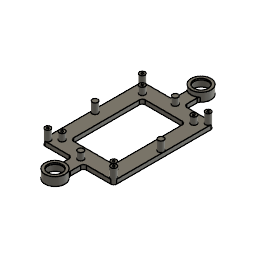
Waterproof box inset (Autodesk Fusion 360 design; units mm, degrees)
Autodesk Fusion 360 part; units mm, degrees
note: some values were not read from the file. Set by a fixed rule: which sketch regions a step uses.
sketch "Sketch1" plane through (0, 0, 0) normal (0, 1, 0) x (1, 0, 0)
  line L0 (0, 0) -> (-50, 0)
  line L1 (-50, 0) -> (-50, 70)
  line L2 (-50, 70) -> (0, 70)
  line L3 (0, 70) -> (0, 0)
  line L4 (-50, 0) -> (-48, 0)
  line L5 (-48, 0) -> (-48, 2)
  line L6 (-48, 2) -> (-50, 2)
  line L7 (-50, 2) -> (-50, 0)
  circle A0 centre (-48, 2) radius 2
  circle A1 centre (-48, 68) radius 2
  circle A2 centre (-2, 68) radius 2
  circle A3 centre (-2, 2) radius 2
  circle A4 centre (-25, 2) radius 2
  circle A5 centre (-25, 68) radius 2
  circle A6 centre (-48, 35) radius 2
  circle A7 centre (-2, 35) radius 2
  line L8 (-23, 68) -> (-23, 70)
  line L9 (-27, 68) -> (-27, 70)
  line L10 (-48, 37) -> (-50, 37)
  line L11 (-48, 33) -> (-50, 33)
  line L12 (-2, 37) -> (0, 37)
  line L13 (-2, 33) -> (0, 33)
  line L14 (-27, 2) -> (-27, 0)
  line L15 (-23, 2) -> (-23, 0)
  line L16 (-4, 2) -> (-4, 0)
  line L17 (-2, 4) -> (0, 4)
  line L18 (-46, 2) -> (-46, 0)
  line L19 (-48, 4) -> (-50, 4)
  line L20 (-48, 66) -> (-50, 66)
  line L21 (-46, 68) -> (-46, 70)
  line L22 (-4, 68) -> (-4, 70)
  line L23 (-2, 66) -> (0, 66)
  line L24 (-23, 70) -> (-27, 70)
  line L25 (-27, 0) -> (-23, 0)
  line L26 (-29, 85) -> (-29, 70)
  line L27 (-21, 87.5) -> (-21, 70)
  line L28 (-29, -15) -> (-29, 0)
  line L29 (-21, -15) -> (-21, 0)
  line L30 (-50, 0) -> (-45, 0)
  line L31 (-45, 5) -> (-5, 5)
  line L32 (-5, 5) -> (-5, 65)
  line L33 (-5, 65) -> (-45, 65)
  line L34 (-45, 65) -> (-45, 5)
  circle A8 centre (-43, 7) radius 2
  circle A9 centre (-7, 7) radius 2
  circle A10 centre (-7, 63) radius 2
  circle A11 centre (-43, 63) radius 2
  circle A12 centre (-48, 68) radius 0.75
  circle A13 centre (-43, 63) radius 0.75
  circle A14 centre (-7, 63) radius 0.75
  circle A15 centre (-2, 68) radius 0.75
  circle A16 centre (-7, 7) radius 0.75
  circle A17 centre (-2, 2) radius 0.75
  circle A18 centre (-48, 2) radius 0.75
  circle A19 centre (-43, 7) radius 0.75
  circle A20 centre (-25, -16) radius 5.05
  circle A21 centre (-25, 86) radius 5.05
  line L35 (-40, 60) -> (-10, 60)
  line L36 (-10, 60) -> (-10, 10)
  line L37 (-10, 10) -> (-40, 10)
  line L38 (-40, 10) -> (-40, 60)
  circle A22 centre (-25, 86) radius 7
  circle A23 centre (-25, -16) radius 7
  dimension "d1" = 50
  dimension "d2" = 70
  dimension "d16" = 1.5
  dimension "d17" = 1.5
  dimension "d18" = 1.5
  dimension "d19" = 1.5
  dimension "d20" = 1.5
  dimension "d21" = 1.5
  dimension "d22" = 1.5
  dimension "d23" = 1.5
  dimension "d24" = 10.1
  dimension "d25" = 10.1
  dimension "d33" = 17.5
  constraint horizontal L0
  constraint vertical L1
  constraint horizontal L2
  constraint vertical L3
  constraint coincident L0.start L3.end
  constraint horizontal L4
  constraint vertical L5
  constraint horizontal L6
  constraint vertical L7
  constraint coincident L5.end L6.start
  constraint coincident L6.end A0
  constraint coincident A5 L8.start
  constraint coincident L2 L8.end
  constraint perpendicular L2 L8
  constraint coincident A5 L9.start
  constraint coincident L2 L9.end
  constraint perpendicular L2 L9
  constraint coincident A6 L10.start
  constraint coincident L1 L10.end
  constraint perpendicular L1 L10
  constraint coincident A6 L11.start
  constraint coincident L1 L11.end
  constraint perpendicular L1 L11
  constraint coincident A7 L12.start
  constraint perpendicular L3 L12
  constraint coincident A7 L13.start
  constraint coincident L3 L13.end
  constraint perpendicular L3 L13
  constraint coincident A4 L14.start
  constraint coincident L0 L14.end
  constraint perpendicular L0 L14
  constraint coincident A4 L15.start
  constraint coincident L0 L15.end
  constraint perpendicular L0 L15
  constraint coincident A3 L16.start
  constraint tangent A3 L16
  constraint perpendicular L0 L16
  constraint coincident A3 L17.start
  constraint coincident L3 L17.end
  constraint tangent A3 L17
  constraint perpendicular L3 L17
  constraint coincident A0 L18.start
  constraint coincident L0 L18.end
  constraint perpendicular L0 L18
  constraint coincident L1 L19.end
  constraint perpendicular L1 L19
  constraint coincident A1 L20.start
  constraint coincident L1 L20.end
  constraint tangent A1 L20
  constraint perpendicular L1 L20
  constraint coincident A1 L21.start
  constraint coincident L2 L21.end
  constraint tangent A1 L21
  constraint perpendicular L2 L21
  constraint coincident A2 L22.start
  constraint coincident L2 L22.end
  constraint tangent A2 L22
  constraint perpendicular L2 L22
  constraint coincident A2 L23.start
  constraint coincident L3 L23.end
  constraint tangent A2 L23
  constraint perpendicular L3 L23
  constraint horizontal L24
  constraint horizontal L25
  constraint coincident L2 L26.end
  constraint perpendicular L2 L26
  constraint coincident L2 L27.end
  constraint perpendicular L2 L27
  constraint coincident L0 L28.end
  constraint perpendicular L0 L28
  constraint coincident L0 L29.end
  constraint perpendicular L0 L29
  constraint coincident L0 L30.end
  constraint horizontal L31
  constraint vertical L32
  constraint horizontal L33
  constraint vertical L34
  constraint concentric A1 A12
  constraint concentric A11 A13
  constraint concentric A10 A14
  constraint concentric A2 A15
  constraint concentric A9 A16
  constraint concentric A3 A17
  constraint concentric A0 A18
  constraint concentric A8 A19
  constraint horizontal L35
  constraint vertical L36
  constraint horizontal L37
  constraint vertical L38
  constraint concentric A21 A22
  constraint concentric A20 A23
  measures "d1" distance of L0.start L0.end
  measures "d2" distance of L0.start L2.end
  measures "d16" diameter of A12
  measures "d17" diameter of A13
  measures "d18" diameter of A14
  measures "d19" diameter of A15
  measures "d20" diameter of A16
  measures "d21" diameter of A17
  measures "d22" diameter of A18
  measures "d23" diameter of A19
  measures "d24" diameter of A20
  measures "d25" diameter of A21
  measures "d33" distance of L27.start L27.end
extrude "Extrude1" add sketch "Sketch1" along normal blind 3 contours L0 A3 L16 | L0 L1 L2 L3 A0 A1 A2 A3 A4 A5 A6 A7 L8 L9 L10 L11 L12 L13 L14 L15 L16 L17 L18 L19 L20 L21 L22 L23 L30 | L0 L25 L28 L29 A23 | A3 | L0 A4 L15 L25 | L28 L29 A20 A23 | L28 L29 A20 A23 | L3 A3 L17 | L0 A4 L14 L25 | A4 | L3 A7 L13 | L3 A7 L12 | A7 | L0 A0 L18 L30 | L5 L6 A0 A18 | L5 L6 A0 A18 | L3 A2 L23 | L5 L6 A18 | L5 L6 A18 | L1 A0 L19 | A2 | L2 A2 L22 | L1 A6 L11 | L1 A6 L10 | A6 | L2 L24 L26 L27 A22 | L2 A5 L8 L24 | L26 L27 A21 A22 | L26 L27 A21 A22 | L1 A1 L20 | L2 A5 L9 L24 | A5 | A1 | L2 A1 L21 | L31 L34 A8 | L31 L32 L33 L34 A8 A9 A10 A11 | A8 | L31 L32 A9 | A9 | L33 L34 A11 | A11 | L32 L33 A10 | A10 | A12 | A13 | A14 | A15 | A16 | A17 | A19
extrude "Extrude2" add sketch "Sketch1" along normal blind 10 contours A3 | A7 | L5 L6 A0 A18 | L5 L6 A0 A18 | A2 | A6 | A1
extrude "Extrude3" add sketch "Sketch1" along normal blind 8 contours A4 | A5 | A8 | A9 | A11 | A10
fillet "Fillet1" radius 2 12 edges at (-29, 1.5, -70) (-21, 1.5, -70) (-21, 1.5, 0) (-29, 1.5, 0) (-10, 1.5, -60) (-10, 1.5, -10) (-40, 1.5, -10) (-40, 1.5, -60) (-29, 1.5, 10.2554) (-21, 1.5, 10.2554) (-29, 1.5, -80.2554) (-21, 1.5, -80.2554)
extrude "Extrude4" add sketch "Sketch1" along normal blind 6 contours L28 L29 A20 A23 | L28 L29 A20 A23 | L26 L27 A21 A22 | L26 L27 A21 A22
chamfer "Chamfer1" distance 5 distance2 1 2 edges at (-29.7083, 0, -87.8262) (-29.7083, 0, 14.1738) measured on face at (-19.9751, 2, -86.5028) measured on face at (-19.9751, 2, 15.4972)
